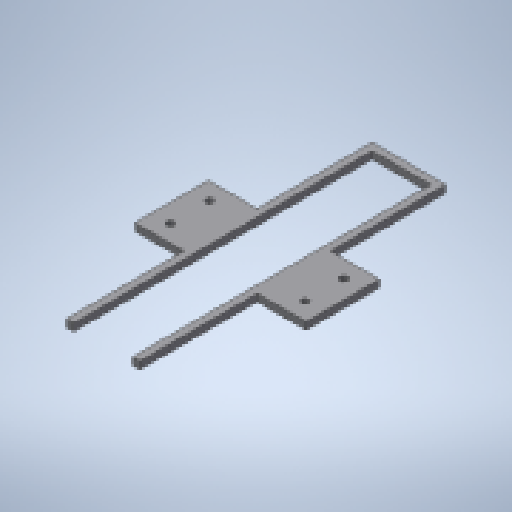
# Autodesk Inventor part: 电池仓
Saved by Autodesk Inventor 2025.2 (Build 292293000, 293)
## iProperties
Created: 2025-10-23
Part Number: 电池仓
Material: 常规
Document SubType Name: Modeling
Designer: BO‘S_SLAVE
Density: 1 g/cm^3
Appearance: 默认
Author: BO‘S_SLAVE
Autodesk Inventor part; units mm, degrees
ref_plane "YZ Plane" through (0, 0, 0) normal (1, 0, 0) x (0, 1, 0)
ref_plane "XZ Plane" through (0, 0, 0) normal (0, 1, 0) x (-1, 0, 0)
ref_plane "XY Plane" through (0, 0, 0) normal (0, 0, 1) x (1, 0, 0)
sketch "草图1" plane through (0, 0, 0) normal (0, 1, 0) x (-1, 0, 0)
  line L0 (-15, -62) -> (15, -62)
  line L1 (15, -62) -> (15, 63)
  line L2 (15, 63) -> (-15, 63)
  line L3 (-15, 63) -> (-15, -62)
  line L4 (12, 59) -> (-12, 59)
  line L5 (-12, 59) -> (-12, -59)
  line L6 (-12, -59) -> (12, -59)
  line L7 (12, -59) -> (12, 59)
  line L8 (-12, 59) -> (-12, 63)
  line L9 (12, 59) -> (12, 63)
  line L10 (-12, 0) -> (12, 0)
  line L11 (0, -59) -> (0, 59)
  circle A0 centre (-27, -8) radius 1.55
  circle A1 centre (-27, 8) radius 1.55
  circle A2 centre (27, -8) radius 1.55
  circle A3 centre (27, 8) radius 1.55
  line L12 (-15, -15) -> (-32, -15)
  line L13 (-32, -15) -> (-32, 15)
  line L14 (-32, 15) -> (-15, 15)
  line L15 (-15, 15) -> (-15, -15)
  line L16 (15, -15) -> (32, -15)
  line L17 (32, -15) -> (32, 15)
  line L18 (32, 15) -> (15, 15)
  line L19 (15, 15) -> (15, -15)
  point P0 (0, 0)
  point P1 (0, 0)
  point P2 (15, 15)
  point P3 (-15, 15)
  dimension "d20" = 125
  dimension "d22" = 24
  dimension "d23" = 3
  dimension "d25" = 118
  dimension "d26" = 3
  dimension "d27" = 3
  dimension "d28" = 30
  dimension "d29" = 30
  dimension "d31" = 7
  dimension "d32" = 17
  dimension "d33" = 17
  dimension "d34" = 3.1
  dimension "d35" = 3.1
  dimension "d36" = 3.1
  dimension "d37" = 3.1
  dimension "d40" = 7
  dimension "d41" = 7
  dimension "d44" = 7
  dimension "d45" = 15
  dimension "d46" = 27
  dimension "d47" = 27
  dimension "d48" = 27
  dimension "d49" = 27
  constraints: 40 end point, 8 parallel, 6 perpendicular, 5 midpoint, 5 point on line, 4 centre point, 4 horizontal, 1 coincident
  measures "d20" distance between parallel lines of L2 L0
  measures "d22" distance between parallel lines of L5 L7
  measures "d23" distance between parallel lines of L6 L0
  measures "d25" distance between parallel lines of L6 L4
  measures "d26" distance between parallel lines of L1 L7
  measures "d27" distance between parallel lines of L3 L5
  measures "d28" distance between parallel lines of L14 L12
  measures "d29" distance between parallel lines of L18 L16
  measures "d31" distance from line of A2.centre L16
  measures "d32" distance between parallel lines of L3 L13
  measures "d33" distance between parallel lines of L1 L17
  measures "d34" diameter of A0
  measures "d35" diameter of A1
  measures "d36" diameter of A3
  measures "d37" diameter of A2
  measures "d40" distance from line of L18 A3.centre
  measures "d41" distance from line of L14 A1.centre
  measures "d44" distance from line of L12 A0.centre
  measures "d45" distance between parallel lines of L10 L12
  measures "d46" distance from line of L11 A2.centre
  measures "d47" distance from line of L11 A0.centre
  measures "d48" distance from line of L11 A1.centre
  measures "d49" distance from line of A3.centre L11
extrude "拉伸1" add sketch "草图1" along normal blind 3 contours L3 L2 L8 L5 L6 L7 L9 L1 L0 | L12 L13 L14 L3 | L1 L18 L17 L16
extrude "拉伸2" add sketch "草图1" against normal blind 31 contours L3 L2 L8 L5 L6 L7 L9 L1 L0
sketch "草图2" plane through (0, -31, 0) normal (0, -1, 0) x (1, 0, 0)
  line L0 (-15, 63) -> (-15, -62) projected
  line L1 (-15, -62) -> (15, -62) projected
  line L2 (15, -62) -> (15, 63) projected
  line L3 (15, 63) -> (12, 63) projected
  line L4 (12, 63) -> (12, -59) projected
  line L5 (12, -59) -> (-12, -59) projected
  line L6 (-12, -59) -> (-12, 63) projected
  line L7 (-12, 63) -> (-15, 63) projected
  line L8 (12, 63) -> (-12, 63)
  point P0 (0, 0)
  constraints: 2 end point, 1 horizontal
extrude "拉伸3" add sketch "草图2" along normal blind 3
fillet "圆角1" radius 5 4 edges at (0, -34, -62) (-15, -34, 0.5) (15, -34, 0.5) (0, -34, 63)
fillet "圆角2" radius 3 8 edges at (13.5355, -32.5355, 61.5355) (15, -13, 63) (-13.5355, -32.5355, 61.5355) (-15, -13, 63) (13.5355, -32.5355, -60.5355) (15, -13, -62) (-13.5355, -32.5355, -60.5355) (-15, -13, -62)
fillet "圆角3" radius 3 6 edges at (32, 0, 0) (23.5, 0, 15) (23.5, 0, -15) (-23.5, 0, -15) (-32, 0, 0) (-23.5, 0, 15)
